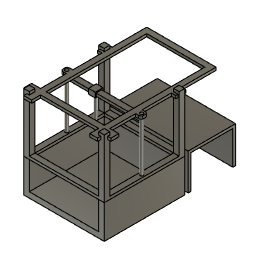
Trolley v7 (Autodesk Fusion 360 design; units mm, degrees)
Autodesk Fusion 360 part; units mm, degrees
sketch "Sketch1" plane through (0, 0, 0) normal (0, 0, 1) x (1, 0, 0)
  line L0 (0, 0) -> (720, 0)
  line L1 (720, 0) -> (720, 720)
  line L2 (720, 720) -> (0, 720)
  line L3 (0, 720) -> (0, 0)
  dimension "d1" = 720
  dimension "d2" = 720
  constraint horizontal L0
  constraint vertical L1
  constraint horizontal L2
  constraint vertical L3
  constraint coincident L0.start L3.end
  measures "d1" distance of L0.start L0.end
  measures "d2" distance of L0.start L2.end
extrude "Extrude1" add sketch "Sketch1" along normal blind 300 makes body 1
shell "Shell1" thickness 50 removed faces 0 bodies 1
sketch "Sketch2" plane through (0, 0, 300) normal (0, 0, 1) x (-1, 0, 0)
  line L0 (0, -720) -> (0, 0)
  line L1 (0, 0) -> (-720, 0)
  line L2 (-720, 0) -> (-720, -720)
  line L3 (-720, -720) -> (0, -720)
  line L4 (-50, -670) -> (-670, -670)
  line L5 (-670, -670) -> (-670, -50)
  line L6 (-670, -50) -> (-50, -50)
  line L7 (-50, -50) -> (-50, -670)
  dimension "d6" = 50
  dimension "d7" = 50
  dimension "d8" = 50
  dimension "d9" = 50
  constraint horizontal L4
  constraint vertical L5
  constraint horizontal L6
  constraint vertical L7
  measures "d6" distance of L2 L5
  measures "d7" distance of L3 L4
  measures "d8" distance of L0 L7
  measures "d9" distance of L1 L6
extrude "Extrude2" cut sketch "Sketch2" against normal blind 100 contours L4 L5 L6 L7 bodies 1
sketch "Sketch3" plane through (0, 0, 0) normal (0, 0, 1) x (1, 0, 0)
  line L0 (0, 0) -> (720, 0)
  line L1 (720, 0) -> (720, 720)
  line L2 (720, 720) -> (0, 720)
  line L3 (0, 720) -> (0, 0)
  line L4 (50, 670) -> (670, 670)
  line L5 (670, 670) -> (670, 50)
  line L6 (670, 50) -> (50, 50)
  line L7 (50, 50) -> (50, 670)
  dimension "d12" = 720
  dimension "d13" = 720
  dimension "d14" = 50
  dimension "d15" = 50
  dimension "d16" = 50
  dimension "d17" = 50
  constraint horizontal L0
  constraint vertical L1
  constraint horizontal L2
  constraint vertical L3
  constraint coincident L0.start L3.end
  constraint horizontal L4
  constraint vertical L5
  constraint horizontal L6
  constraint vertical L7
  measures "d12" distance of L0.start L0.end
  measures "d13" distance of L0.start L2.end
  measures "d14" distance of L2 L4
  measures "d15" distance of L1 L5
  measures "d16" distance of L3 L7
  measures "d17" distance of L0 L6
extrude "Extrude3" add sketch "Sketch3" along normal blind 25 separate body makes body 2
sketch "Sketch4" plane through (0, 0, 25) normal (0, 0, 1) x (-1, 0, 0)
  line L0 (-670, -50) -> (-50, -50)
  line L1 (-50, -50) -> (-50, -670)
  line L2 (-50, -670) -> (-670, -670)
  line L3 (-670, -670) -> (-670, -50)
  line L4 (0, -720) -> (0, 0)
  line L5 (0, 0) -> (-720, 0)
  line L6 (-720, 0) -> (-720, -720)
  line L7 (-720, -720) -> (0, -720)
  line L8 (-50, -360) -> (-670, -360) construction
  line L9 (-670, -360) -> (-720, -360) construction
  circle A0 centre (-695, -360) radius 15
  dimension "d20" = 30
  constraint midpoint L1 L8.start
  constraint midpoint L3 L8.end
  constraint midpoint L6 L9.end
  constraint midpoint L9 A0.centre
  measures "d20" diameter of A0
extrude "Extrude4" add sketch "Sketch4" along normal blind 500 separate body contours A0 makes body 3
ref_plane "WorkPlane1" through (360, 360, 12.5) normal (1, 0, 0) x (0, 1, 0)
mirror "Mirror1" about plane through (360, 360, 12.5) normal (1, 0, 0) of bodies 3 makes body 4
sketch "Sketch5" plane through (0, 0, 525) normal (0, 0, 1) x (-1, 0, 0)
  circle A0 centre (-695, -360) radius 15
  line L0 (-670, -50) -> (-50, -50)
  line L1 (-50, -50) -> (-50, -670)
  line L2 (-50, -670) -> (-670, -670)
  line L3 (-670, -670) -> (-670, -50)
  line L4 (0, -720) -> (0, 0)
  line L5 (0, 0) -> (-720, 0)
  line L6 (-720, 0) -> (-720, -720)
  line L7 (-720, -720) -> (0, -720)
  line L8 (-50, -670) -> (-670, -670)
  line L9 (-670, -50) -> (-50, -50)
  line L10 (-620, -100) -> (-100, -100)
  line L11 (-100, -100) -> (-100, -620)
  line L12 (-100, -620) -> (-620, -620)
  line L13 (-620, -620) -> (-620, -100)
  line L14 (-695, -390) -> (-670, -390)
  line L15 (-695, -360) -> (-725, -360) construction
  line L16 (-695, -330) -> (-670, -330)
  arc A1 (-695, -330) -> (-695, -390) centre (-695, -360) ccw
  line L17 (-670, -670) -> (-670, -390)
  line L18 (-670, -330) -> (-670, -50)
  line L19 (-360, -50) -> (-360, -720) construction
  line L20 (-25, -390) -> (-50, -390)
  arc A2 (-25, -390) -> (-25, -330) centre (-25, -360) ccw
  circle A3 centre (-25, -360) radius 15
  line L21 (-25, -330) -> (-50, -330)
  line L22 (-50, -50) -> (-50, -330)
  line L23 (-50, -390) -> (-50, -670)
  dimension "d26" = 60
  constraint horizontal L8
  constraint vertical L17
  constraint horizontal L9
  constraint vertical L22
  constraint coincident L0.start L3.end
  constraint coincident L1.end L2.start
  constraint concentric A0 A1
  constraint tangent L14 A1
  constraint horizontal L14
  constraint coincident L3 L14.end
  constraint coincident A0.centre L15.start
  constraint coincident L15.end A1
  constraint perpendicular L6 L15
  constraint symmetric L14.start L15 L16.start
  constraint symmetric L14.end L15 L16.end
  constraint collinear L17 L18
  constraint midpoint L0 L19.start
  constraint midpoint L7 L19.end
  constraint symmetric A0 L19 A3
  constraint symmetric L14.start L19 L20.start
  constraint symmetric L14.end L19 L20.end
  constraint symmetric L16.start L19 A2.end
  constraint symmetric L16.end L19 L21.end
  constraint symmetric A1 L19 A2
  constraint collinear L22 L23
  measures "d26" diameter of A1
extrude "Extrude1'" add sketch "Sketch5" against normal blind 25 separate body contours L0 L1 L2 L3 L8 L9 L17 L18 L22 L23 | L3 L6 L14 L16 A1 | L1 L4 L20 A2 L21 makes body 5 in component "Z axis"
copy_body "Body->Comp1" bodies 1 removing the originals makes body 6 in component "Container"
copy_body "Body->Comp2" bodies 2 removing the originals makes body 7 in component "Frame"
copy_body "Body->Comp3" bodies 3 removing the originals makes body 8 in component "Guide 1"
copy_body "Body->Comp4" bodies 4 removing the originals makes body 9 in component "Guide 2"
sketch "Sketch6" plane through (0, 0, 0) normal (0, 0, -1) x (1, 0, 0)
  line L0 (50, -50) -> (670, -50)
  line L1 (670, -50) -> (670, -670)
  line L2 (670, -670) -> (50, -670)
  line L3 (50, -670) -> (50, -50)
  line L4 (0, 0) -> (0, -720)
  line L5 (0, -720) -> (720, -720)
  line L6 (720, -720) -> (720, 0)
  line L7 (720, 0) -> (0, 0)
  circle A0 centre (695, -360) radius 15
extrude "Extrude1''" cut sketch "Sketch6" against normal blind 25 contours A0 bodies 7 in component "Frame"
mirror "Mirror1'" about plane through (360, 360, 12.5) normal (1, 0, 0) of "Extrude1''" in component "Frame"
sketch "Sketch7" plane through (0, 0, 0) normal (0, 1, 0) x (1, 0, 0)
  line L0 (670, -500) -> (50, -500)
  line L1 (50, -500) -> (50, -475)
  line L2 (50, -475) -> (670, -475)
  line L3 (670, -475) -> (670, -500)
  line L4 (50, -475) -> (50, -390) construction
  line L5 (670, -475) -> (670, -400) construction
  line L6 (70, -450) -> (650, -450)
  line L7 (670, -450) -> (670, -425)
  line L8 (670, -425) -> (50, -425)
  line L9 (50, -425) -> (50, -450)
  line L10 (50, -450) -> (50, -475)
  line L11 (70, -450) -> (70, -475)
  line L12 (360, -425) -> (360, -550) construction
  line L13 (650, -450) -> (650, -475)
  line L14 (670, -450) -> (670, -475)
  dimension "d47" = 25
  constraint coincident L1.end L2.start
  constraint perpendicular L2 L4
  constraint coincident L2.end L3.start
  constraint perpendicular L2 L5
  constraint horizontal L6
  constraint vertical L7
  constraint horizontal L8
  constraint vertical L9
  constraint coincident L4 L9.end
  constraint coincident L2 L11.end
  constraint perpendicular L2 L11
  constraint midpoint L8 L12.start
  constraint perpendicular L6 L12
  constraint symmetric L9.end L12 L7.start
  constraint symmetric L1.end L12 L2.end
  constraint symmetric L6.start L12 L6.end
  constraint symmetric L11.end L12 L13.end
  measures "d47" distance of L9.end L8.end
extrude "Extrude5" add sketch "Sketch7" along normal blind 50 separate body contours L2 L6 L7 L8 L9 L10 L11 L13 L14 makes body 10
sketch "Sketch8" plane through (670, 0, 0) normal (1, 0, 0) x (0, 1, 0)
  line L0 (0, 475) -> (0, 425)
  line L1 (0, 425) -> (50, 425)
  line L2 (50, 425) -> (50, 475)
  line L3 (50, 475) -> (0, 475)
  line L4 (0, 450) -> (50, 450)
  line L5 (0, 450) -> (50, 450)
  line L6 (50, 425) -> (0, 425)
  line L7 (0, 450) -> (0, 425)
  line L8 (50, 450) -> (50, 425)
  line L9 (-10, 460) -> (60, 460)
  line L10 (60, 460) -> (60, 415)
  line L11 (60, 415) -> (-10, 415)
  line L12 (-10, 460) -> (-10, 415)
  dimension "d50" = -10
  constraint coincident L4.start L5.start
  constraint coincident L4.end L5.end
  constraint coincident L1.end L2.start
  constraint coincident L0.end L1.start
extrude "Extrude1'''" add sketch "Sketch8" against normal blind 60 separate body contours L0 L1 L2 L6 L7 L8 L9 L10 L11 L12 | L0 L2 L4 L5 L9 makes body 11 in component "X axis"
copy_body "Body->Comp5" bodies 10 removing the originals makes body 12 in component "Y axis"
sketch "Sketch9" plane through (60.5346, 64.5547, 417.5) normal (0, 0, -1) x (1, 0, 0)
  line L0 (329.4654, -590.4453) -> (329.4654, -520.4453)
  line L1 (329.4654, -520.4453) -> (269.4654, -520.4453)
  line L2 (269.4654, -520.4453) -> (269.4654, -590.4453)
  line L3 (269.4654, -590.4453) -> (329.4654, -590.4453)
  line L4 (329.4654, -590.4453) -> (269.4654, -520.4453) construction
  line L5 (329.4654, -520.4453) -> (269.4654, -590.4453) construction
  circle A0 centre (299.4654, -555.4453) radius 12.5
  dimension "d65" = 25
  constraint coincident L0.start L3.end
  constraint coincident L1.end L2.start
  constraint coincident L0.end L1.start
  constraint coincident L2.end L3.start
  constraint midpoint L4 A0.centre
  measures "d65" diameter of A0
extrude "Extrude2'" add sketch "Sketch9" along normal blind 200 contours A0 sketch seen with x (1, 0, 0) y (0, 1, 0) z (0, 0, 1) at (280, -595, -2.5) bodies 11 in component "X axis"
sketch "Sketch10" plane through (720, 0, 0) normal (1, 0, 0) x (0, 1, 0)
  line L0 (0, -300) -> (720, -300)
  line L1 (720, -300) -> (720, 0)
  line L2 (720, 0) -> (0, 0)
  line L3 (0, 0) -> (0, -300)
  line L4 (750, 25) -> (1175, 25)
  line L5 (1175, 25) -> (1175, -300)
  line L6 (750, -300) -> (750, 25)
  line L7 (775, -300) -> (775, 0)
  line L8 (775, 0) -> (1150, 0)
  line L9 (1150, 0) -> (1150, -300)
  line L10 (1175, -300) -> (1150, -300)
  line L11 (775, -300) -> (750, -300)
  constraint horizontal L4
  constraint vertical L5
  constraint horizontal L10
  constraint vertical L6
  constraint coincident L7.start L10
  constraint perpendicular L7 L10
  constraint perpendicular L7 L8
  constraint perpendicular L9 L10
  constraint collinear L10 L11
extrude "Extrude6" add sketch "Sketch10" against normal blind 700 separate body contours L4 L5 L6 L7 L8 L9 L10 L11 makes body 13
sketch "Sketch11" plane through (0, 0, 500) normal (0, 0, 1) x (-1, 0, 0)
  circle A0 centre (-695, -360) radius 15
  line L0 (-100, -620) -> (-620, -620)
  line L1 (-620, -620) -> (-620, -100)
  line L2 (-620, -100) -> (-100, -100)
  line L3 (-100, -100) -> (-100, -620)
  circle A1 centre (-25, -360) radius 15
  arc A2 (-25, -390) -> (0, -376.5831) centre (-25, -360) ccw
  line L4 (0, -376.5831) -> (0, -343.4169)
  arc A3 (0, -343.4169) -> (-25, -330) centre (-25, -360) ccw
  line L5 (-25, -330) -> (-50, -330)
  line L6 (-50, -330) -> (-50, -50)
  line L7 (-50, -50) -> (-670, -50)
  line L8 (-670, -50) -> (-670, -330)
  line L9 (-670, -330) -> (-695, -330)
  arc A4 (-695, -330) -> (-720, -343.4169) centre (-695, -360) ccw
  line L10 (-720, -343.4169) -> (-720, -376.5831)
  arc A5 (-720, -376.5831) -> (-695, -390) centre (-695, -360) ccw
  line L11 (-695, -390) -> (-670, -390)
  line L12 (-670, -390) -> (-670, -670)
  line L13 (-670, -670) -> (-50, -670)
  line L14 (-50, -670) -> (-50, -390)
  line L15 (-50, -390) -> (-25, -390)
  line L16 (-670, -670) -> (-670, -1050)
  line L17 (-670, -1050) -> (-50, -1050)
  line L18 (-50, -1050) -> (-50, -670)
  line L19 (-620, -620) -> (-620, -1000)
  line L20 (-620, -1000) -> (-100, -1000)
  line L21 (-100, -1000) -> (-100, -620)
  constraint coincident L12.end L13.start
  constraint perpendicular L13 L16
  constraint perpendicular L16 L17
  constraint coincident L13.end L14.start
  constraint perpendicular L13 L18
  constraint coincident L0.end L1.start
  constraint perpendicular L13 L19
  constraint perpendicular L1 L20
  constraint coincident L0.start L3.end
  constraint perpendicular L0 L21
extrude "Extrude2''" add sketch "Sketch11" against normal blind 25 contours L13 L16 L17 L18 L19 L20 L21 sketch seen with x (1, 0, 0) y (0, 1, 0) z (0, 0, 1) at (0, 0, 25) bodies 5 in component "Z axis"
sketch "Sketch12" plane through (0, 0, 0) normal (0, -1, 0) x (1, 0, 0)
  line L0 (0, -300) -> (720, -300)
  line L1 (720, -300) -> (720, 0)
  line L2 (720, 0) -> (0, 0)
  line L3 (0, 0) -> (0, -300)
move_face "OffsetFaces1" offset -500 1 faces at (463.3333, 50, 216.6667) on bodies 6 in component "Container"
sketch "Sketch13" plane through (0, 0, 25) normal (0, 0, 1) x (-1, 0, 0)
  circle A0 centre (-25, -360) radius 15
  circle A1 centre (-695, -360) radius 15
  line L0 (-670, -50) -> (-50, -50)
  line L1 (-50, -50) -> (-50, -670)
  line L2 (-50, -670) -> (-670, -670)
  line L3 (-670, -670) -> (-670, -50)
  line L4 (0, -720) -> (0, 0)
  line L5 (0, 0) -> (-720, 0)
  line L6 (-720, 0) -> (-720, -720)
  line L7 (-720, -720) -> (0, -720)
  line L8 (0, 0) -> (-50, 0)
  line L9 (-50, 0) -> (-50, -50)
  line L10 (-50, -50) -> (0, -50)
  line L11 (0, -50) -> (0, 0)
  constraint horizontal L8
  constraint vertical L9
  constraint horizontal L10
  constraint vertical L11
  constraint coincident L0.end L1.start
  constraint coincident L4.end L5.start
extrude "Extrude2'''" add sketch "Sketch13" along normal blind 500 contours L4 L5 L8 L9 L10 L11 bodies 7 in component "Frame"
sketch "Sketch14" plane through (0, 0, 500) normal (0, 0, 1) x (-1, 0, 0)
  line L0 (-50, -1050) -> (-50, -390)
  line L1 (-50, -390) -> (-25, -390)
  arc A0 (-25, -390) -> (0, -376.5831) centre (-25, -360) ccw
  line L2 (0, -376.5831) -> (0, -343.4169)
  arc A1 (0, -343.4169) -> (-25, -330) centre (-25, -360) ccw
  line L3 (-25, -330) -> (-50, -330)
  line L4 (-50, -330) -> (-50, -50)
  line L5 (-50, -50) -> (-670, -50)
  line L6 (-670, -50) -> (-670, -330)
  line L7 (-670, -330) -> (-695, -330)
  arc A2 (-695, -330) -> (-720, -343.4169) centre (-695, -360) ccw
  line L8 (-720, -343.4169) -> (-720, -376.5831)
  arc A3 (-720, -376.5831) -> (-695, -390) centre (-695, -360) ccw
  line L9 (-695, -390) -> (-670, -390)
  line L10 (-670, -390) -> (-670, -1050)
  line L11 (-670, -1050) -> (-50, -1050)
  circle A4 centre (-695, -360) radius 15
  line L12 (-100, -620) -> (-620, -620)
  line L13 (-620, -620) -> (-620, -100)
  line L14 (-620, -100) -> (-100, -100)
  line L15 (-100, -100) -> (-100, -620)
  circle A5 centre (-25, -360) radius 15
  line L16 (-100, -670) -> (-100, -1000)
  line L17 (-100, -1000) -> (-620, -1000)
  line L18 (-620, -1000) -> (-620, -670)
  line L19 (-620, -670) -> (-100, -670)
  line L20 (-50, -100) -> (30, -100)
  line L21 (30, -100) -> (30, -30)
  line L22 (30, -30) -> (0, -30)
  line L23 (0, -30) -> (0, -50)
  line L24 (0, -50) -> (-50, -50)
  line L25 (-50, -50) -> (-100, -100) construction
  line L26 (-100, -50) -> (-100, 30)
  line L27 (-100, 30) -> (-30, 30)
  line L28 (-30, 30) -> (-30, 0)
  line L29 (-50, 0) -> (-50, -50)
  line L30 (-30, 0) -> (-50, 0)
  line L31 (-360, -50) -> (-360, -250) construction
  line L32 (-670, -100) -> (-750, -100)
  line L33 (-750, -100) -> (-750, -30)
  line L34 (-750, -30) -> (-720, -30)
  line L35 (-720, -30) -> (-720, -50)
  line L36 (-720, -50) -> (-670, -50)
  line L37 (-670, 0) -> (-670, -50)
  line L38 (-690, 0) -> (-670, 0)
  line L39 (-690, 30) -> (-690, 0)
  line L40 (-620, 30) -> (-690, 30)
  line L41 (-620, -50) -> (-620, 30)
  constraint coincident L4 L20.start
  constraint perpendicular L4 L20
  constraint perpendicular L20 L21
  constraint perpendicular L21 L22
  constraint perpendicular L22 L23
  constraint coincident L4.end L5.start
  constraint perpendicular L4 L24
  constraint coincident L14.end L15.start
  constraint symmetric L20.start L25 L26.start
  constraint symmetric L20.end L25 L26.end
  constraint symmetric L21.end L25 L27.end
  constraint symmetric L22.end L25 L28.end
  constraint symmetric L23.end L25 L29.start
  constraint symmetric L4.end L25 L5.start
  constraint midpoint L5 L31.start
  constraint perpendicular L5 L31
  constraint symmetric L20.start L31 L32.start
  constraint symmetric L20.end L31 L32.end
  constraint symmetric L21.end L31 L33.end
  constraint symmetric L22.end L31 L34.end
  constraint symmetric L23.end L31 L35.end
  constraint symmetric L4.end L31 L5.end
  constraint symmetric L26.start L31 L41.start
  constraint symmetric L26.end L31 L40.start
  constraint symmetric L27.end L31 L39.start
  constraint symmetric L28.end L31 L38.start
  constraint symmetric L29.start L31 L37.start
extrude "Extrude3'" add sketch "Sketch14" against normal blind 25 contours L4 L20 L21 L22 L23 L24 | L5 L26 L27 L28 L29 L30 sketch seen with x (1, 0, 0) y (0, 1, 0) z (0, 0, 1) at (0, 0, 25) bodies 5 in component "Z axis"
sketch "Sketch15" plane through (0, 0, 25) normal (0, 0, 1) x (-1, 0, 0)
  line L0 (-50, -50) -> (-50, 0)
  line L1 (-50, 0) -> (-720, 0)
  line L2 (-720, 0) -> (-720, -720)
  line L3 (-720, -720) -> (0, -720)
  line L4 (0, -720) -> (0, -50)
  line L5 (0, -50) -> (-50, -50)
  line L6 (-50, -50) -> (-50, -670)
  line L7 (-50, -670) -> (-670, -670)
  line L8 (-670, -670) -> (-670, -50)
  line L9 (-670, -50) -> (-50, -50)
  circle A0 centre (-25, -360) radius 15
  circle A1 centre (-695, -360) radius 15
  line L10 (-720, 0) -> (-670, 0)
  line L11 (-670, 0) -> (-670, -50)
  line L12 (-670, -50) -> (-720, -50)
  line L13 (-720, -50) -> (-720, 0)
  dimension "d81" = 50
  dimension "d82" = 50
  constraint horizontal L10
  constraint vertical L11
  constraint horizontal L12
  constraint vertical L13
  constraint coincident L1.end L2.start
  measures "d81" distance of L1.end L10.end
  measures "d82" distance of L1.end L12.end
extrude "Extrude3''" add sketch "Sketch15" along normal blind 500 contours L1 L2 L10 L11 L12 L13 bodies 7 in component "Frame"
extrude "Extrude4'" add sketch "Sketch14" against normal blind 25 contours L6 L32 L33 L34 L35 L36 | L5 L37 L38 L39 L40 L41 sketch seen with x (1, 0, 0) y (0, 1, 0) z (0, 0, 1) at (0, 0, 25) bodies 5 in component "Z axis"
sketch "Sketch16" plane through (0, 0, 25) normal (0, 0, 1) x (-1, 0, 0)
  line L0 (-670, -50) -> (-720, -50)
  line L1 (-720, -50) -> (-720, -720)
  line L2 (-720, -720) -> (0, -720)
  line L3 (0, -720) -> (0, -50)
  line L4 (0, -50) -> (-50, -50)
  line L5 (-50, -50) -> (-50, -670)
  line L6 (-50, -670) -> (-670, -670)
  line L7 (-670, -670) -> (-670, -50)
  circle A0 centre (-25, -360) radius 15
  circle A1 centre (-695, -360) radius 15
  line L8 (-720, -720) -> (-670, -720)
  line L9 (-670, -720) -> (-670, -670)
  line L10 (-670, -670) -> (-720, -670)
  line L11 (-720, -670) -> (-720, -720)
  dimension "d87" = 50
  dimension "d88" = 50
  constraint horizontal L8
  constraint vertical L9
  constraint horizontal L10
  constraint vertical L11
  constraint coincident L1.end L2.start
  measures "d87" distance of L1.end L8.end
  measures "d88" distance of L1.end L10.end
extrude "Extrude4''" add sketch "Sketch16" along normal blind 500 contours L1 L2 L8 L9 L10 L11 bodies 7 in component "Frame"
sketch "Sketch17" plane through (0, 0, 500) normal (0, 0, 1) x (-1, 0, 0)
  line L0 (-50, -1050) -> (-50, -390)
  line L1 (-50, -390) -> (-25, -390)
  arc A0 (-25, -390) -> (0, -376.5831) centre (-25, -360) ccw
  line L2 (0, -376.5831) -> (0, -343.4169)
  arc A1 (0, -343.4169) -> (-25, -330) centre (-25, -360) ccw
  line L3 (-25, -330) -> (-50, -330)
  line L4 (-50, -330) -> (-50, -100)
  line L5 (-50, -100) -> (30, -100)
  line L6 (30, -100) -> (30, -30)
  line L7 (30, -30) -> (0, -30)
  line L8 (0, -30) -> (0, -50)
  line L9 (0, -50) -> (-50, -50)
  line L10 (-50, -50) -> (-50, 0)
  line L11 (-50, 0) -> (-30, 0)
  line L12 (-30, 0) -> (-30, 30)
  line L13 (-30, 30) -> (-100, 30)
  line L14 (-100, 30) -> (-100, -50)
  line L15 (-100, -50) -> (-620, -50)
  line L16 (-620, -50) -> (-620, 30)
  line L17 (-620, 30) -> (-690, 30)
  line L18 (-690, 30) -> (-690, 0)
  line L19 (-690, 0) -> (-670, 0)
  line L20 (-670, 0) -> (-670, -50)
  line L21 (-670, -50) -> (-720, -50)
  line L22 (-720, -50) -> (-720, -30)
  line L23 (-720, -30) -> (-750, -30)
  line L24 (-750, -30) -> (-750, -100)
  line L25 (-750, -100) -> (-670, -100)
  line L26 (-670, -100) -> (-670, -330)
  line L27 (-670, -330) -> (-695, -330)
  arc A2 (-695, -330) -> (-720, -343.4169) centre (-695, -360) ccw
  line L28 (-720, -343.4169) -> (-720, -376.5831)
  arc A3 (-720, -376.5831) -> (-695, -390) centre (-695, -360) ccw
  line L29 (-695, -390) -> (-670, -390)
  line L30 (-670, -390) -> (-670, -1050)
  line L31 (-670, -1050) -> (-50, -1050)
  circle A4 centre (-695, -360) radius 15
  line L32 (-100, -620) -> (-620, -620)
  line L33 (-620, -620) -> (-620, -100)
  line L34 (-620, -100) -> (-100, -100)
  line L35 (-100, -100) -> (-100, -620)
  circle A5 centre (-25, -360) radius 15
  line L36 (-100, -670) -> (-100, -1000)
  line L37 (-100, -1000) -> (-620, -1000)
  line L38 (-620, -1000) -> (-620, -670)
  line L39 (-620, -670) -> (-100, -670)
  line L40 (-670, -740) -> (-710, -740)
  line L41 (-710, -740) -> (-710, -720)
  line L42 (-710, -720) -> (-670, -720)
  line L43 (-670, -720) -> (-670, -740)
  line L44 (-720, -670) -> (-720, -720)
  line L45 (-720, -720) -> (-670, -720)
  line L46 (-670, -720) -> (-670, -670)
  line L47 (-670, -670) -> (-720, -670)
  line L48 (-720, -695) -> (-690, -695) construction
  line L49 (-670, -650) -> (-710, -650)
  line L50 (-710, -650) -> (-710, -670)
  line L51 (-710, -670) -> (-670, -670)
  line L52 (-360, -1050) -> (-360, -965.2348) construction
  line L53 (-50, -740) -> (-10, -740)
  line L54 (-10, -740) -> (-10, -720)
  line L55 (-10, -720) -> (-50, -720)
  line L56 (-10, -650) -> (-10, -670)
  line L57 (-50, -650) -> (-10, -650)
  line L58 (-10, -670) -> (-50, -670)
  constraint horizontal L40
  constraint vertical L41
  constraint horizontal L42
  constraint vertical L43
  constraint coincident L30 L40.start
  constraint midpoint L44 L48.start
  constraint perpendicular L44 L48
  constraint symmetric L40.start L48 L49.start
  constraint symmetric L40.end L48 L49.end
  constraint symmetric L41.end L48 L50.end
  constraint symmetric L42.end L48 L46.end
  constraint midpoint L31 L52.start
  constraint perpendicular L37 L52
  constraint symmetric L40.start L52 L53.start
  constraint symmetric L40.end L52 L53.end
  constraint symmetric L41.end L52 L54.end
  constraint symmetric L42.end L52 L55.end
  constraint symmetric L49.start L52 L57.start
  constraint symmetric L49.end L52 L56.start
  constraint symmetric L50.end L52 L56.end
  constraint symmetric L46.end L52 L58.end
extrude "Extrude5'" add sketch "Sketch17" against normal blind 25 contours L30 L40 L41 L42 L43 L45 | L30 L47 L49 L50 L51 sketch seen with x (1, 0, 0) y (0, 1, 0) z (0, 0, 1) at (0, 0, 25) bodies 5 in component "Z axis"
sketch "Sketch18" plane through (0, 0, 25) normal (0, 0, 1) x (-1, 0, 0)
  line L0 (-670, -670) -> (-670, -720)
  line L1 (-670, -720) -> (0, -720)
  line L2 (0, -720) -> (0, -50)
  line L3 (0, -50) -> (-50, -50)
  line L4 (-50, -50) -> (-50, -670)
  line L5 (-50, -670) -> (-670, -670)
  circle A0 centre (-25, -360) radius 15
  line L6 (0, -720) -> (-50, -720)
  line L7 (-50, -720) -> (-50, -670)
  line L8 (-50, -670) -> (0, -670)
  line L9 (0, -670) -> (0, -720)
  dimension "d93" = 50
  dimension "d94" = 50
  constraint horizontal L6
  constraint vertical L7
  constraint horizontal L8
  constraint vertical L9
  constraint coincident L1.end L2.start
  measures "d93" distance of L1.end L6.end
  measures "d94" distance of L1.end L8.end
sketch "Sketch19" plane through (0, 0, 25) normal (0, 0, 1) x (-1, 0, 0)
  line L0 (-670, -670) -> (-670, -720)
  line L1 (-670, -720) -> (0, -720)
  line L2 (0, -720) -> (0, -50)
  line L3 (0, -50) -> (-50, -50)
  line L4 (-50, -50) -> (-50, -670)
  line L5 (-50, -670) -> (-670, -670)
  circle A0 centre (-25, -360) radius 15
  line L6 (0, -720) -> (-50, -720)
  line L7 (-50, -720) -> (-50, -670)
  line L8 (-50, -670) -> (0, -670)
  line L9 (0, -670) -> (0, -720)
  constraint horizontal L6
  constraint vertical L7
  constraint horizontal L8
  constraint vertical L9
  constraint coincident L4.end L5.start
  constraint coincident L1.end L2.start
extrude "Extrude5''" add sketch "Sketch19" along normal blind 500 contours L1 L2 L6 L7 L8 L9 bodies 7 in component "Frame"
extrude "Extrude7" add sketch "Sketch17" against normal blind 25 contours L0 L53 L54 L55 | L0 L56 L57 L58 sketch seen with x (1, 0, 0) y (0, 1, 0) z (0, 0, 1) at (0, 0, 25) bodies 5 in component "Z axis"
sketch "Sketch20" plane through (0, 0, 500) normal (0, 0, 1) x (-1, 0, 0)
  line L0 (-50, -650) -> (-50, -390)
  line L1 (-50, -390) -> (-25, -390)
  arc A0 (-25, -390) -> (0, -376.5831) centre (-25, -360) ccw
  line L2 (0, -376.5831) -> (0, -343.4169)
  arc A1 (0, -343.4169) -> (-25, -330) centre (-25, -360) ccw
  line L3 (-25, -330) -> (-50, -330)
  line L4 (-50, -330) -> (-50, -100)
  line L5 (-50, -100) -> (30, -100)
  line L6 (30, -100) -> (30, -30)
  line L7 (30, -30) -> (0, -30)
  line L8 (0, -30) -> (0, -50)
  line L9 (0, -50) -> (-50, -50)
  line L10 (-50, -50) -> (-50, 0)
  line L11 (-50, 0) -> (-30, 0)
  line L12 (-30, 0) -> (-30, 30)
  line L13 (-30, 30) -> (-100, 30)
  line L14 (-100, 30) -> (-100, -50)
  line L15 (-100, -50) -> (-620, -50)
  line L16 (-620, -50) -> (-620, 30)
  line L17 (-620, 30) -> (-690, 30)
  line L18 (-690, 30) -> (-690, 0)
  line L19 (-690, 0) -> (-670, 0)
  line L20 (-670, 0) -> (-670, -50)
  line L21 (-670, -50) -> (-720, -50)
  line L22 (-720, -50) -> (-720, -30)
  line L23 (-720, -30) -> (-750, -30)
  line L24 (-750, -30) -> (-750, -100)
  line L25 (-750, -100) -> (-670, -100)
  line L26 (-670, -100) -> (-670, -330)
  line L27 (-670, -330) -> (-695, -330)
  arc A2 (-695, -330) -> (-720, -343.4169) centre (-695, -360) ccw
  line L28 (-720, -343.4169) -> (-720, -376.5831)
  arc A3 (-720, -376.5831) -> (-695, -390) centre (-695, -360) ccw
  line L29 (-695, -390) -> (-670, -390)
  line L30 (-670, -390) -> (-670, -650)
  line L31 (-670, -650) -> (-710, -650)
  line L32 (-710, -650) -> (-710, -670)
  line L33 (-710, -670) -> (-670, -670)
  line L34 (-670, -670) -> (-670, -720)
  line L35 (-670, -720) -> (-710, -720)
  line L36 (-710, -720) -> (-710, -740)
  line L37 (-710, -740) -> (-670, -740)
  line L38 (-670, -740) -> (-670, -1050)
  line L39 (-670, -1050) -> (-50, -1050)
  line L40 (-50, -1050) -> (-50, -740)
  line L41 (-50, -740) -> (-10, -740)
  line L42 (-10, -740) -> (-10, -720)
  line L43 (-10, -720) -> (-50, -720)
  line L44 (-50, -720) -> (-50, -670)
  line L45 (-50, -670) -> (-10, -670)
  line L46 (-10, -670) -> (-10, -650)
  line L47 (-10, -650) -> (-50, -650)
  circle A4 centre (-695, -360) radius 15
  line L48 (-100, -620) -> (-620, -620)
  line L49 (-620, -620) -> (-620, -100)
  line L50 (-620, -100) -> (-100, -100)
  line L51 (-100, -100) -> (-100, -620)
  circle A5 centre (-25, -360) radius 15
  line L52 (-100, -670) -> (-100, -1000)
  line L53 (-100, -1000) -> (-620, -1000)
  line L54 (-620, -1000) -> (-620, -670)
  line L55 (-620, -670) -> (-100, -670)
  line L56 (-100, -670) -> (-620, -670)
  line L57 (-620, -670) -> (-620, -620)
  line L58 (-620, -620) -> (-100, -620)
  line L59 (-100, -620) -> (-100, -670)
  constraint horizontal L56
  constraint vertical L57
  constraint horizontal L58
  constraint vertical L59
  constraint coincident L48.end L49.start
  constraint coincident L52.start L55.end
extrude "Extrude8" cut sketch "Sketch20" against normal blind 100 contours L48 L55 L56 L57 L58 L59 sketch seen with x (1, 0, 0) y (0, 1, 0) z (0, 0, 1) at (0, 0, 25) bodies 5 in component "Z axis"
component "Z axis" placed x (1, 0, 0) y (0, 1, 0) z (0, 0, 1) at (0, 0, -25)
component "Container" placed x (1, 0, 0) y (0, 1, 0) z (0, 0, 1) at (0, 0, -300)
component "Frame" placed x (1, 0, 0) y (0, 1, 0) z (0, 0, 1) at (0, 0, 0)
component "Guide 1" placed x (1, 0, 0) y (0, 1, 0) z (0, 0, 1) at (0, 0, -25)
component "Guide 2" placed x (1, 0, 0) y (0, 1, 0) z (0, 0, 1) at (0, 0, -25)
component "X axis" placed x (1, 0, 0) y (0, 1, 0) z (0, 0, 1) at (-383.8326, 362.8376, 2.5)
component "Y axis" placed x (1, 0, 0) y (0, 1, 0) z (0, 0, 1) at (0, 362.8376, 0)
